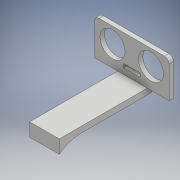
# Autodesk Inventor part: SensorMount
Saved by Autodesk Inventor 2018 (Build 220112000, 112)
## iProperties
Created: 2018-03-20
Part Number: SensorMount
Material: Generic
Document SubType Name: Modeling
Designer: reide
Density: 1 g/cm^3
Appearance: Default
Author: reide
Autodesk Inventor part; units mm, degrees
ref_plane "YZ Plane" through (0, 0, 0) normal (1, 0, 0) x (0, 1, 0)
ref_plane "XZ Plane" through (0, 0, 0) normal (0, 1, 0) x (-1, 0, 0)
ref_plane "XY Plane" through (0, 0, 0) normal (0, 0, 1) x (1, 0, 0)
sketch "Sketch1" plane through (0, 0, 0) normal (1, 0, 0) x (0, 1, 0)
  arc A0 (-24.3967, 0) -> (-49.3967, -25) centre (-24.3967, -25) ccw projected
  line L0 (-10.5765, 0) -> (-24.3967, 0) projected
  line L1 (-10.5765, 0) -> (63.7352, 0) projected
  line L2 (-24.3967, 0) -> (-39.3967, 0)
  line L3 (-39.3967, 0) -> (-39.3967, -5)
  line L4 (-39.3967, 0) -> (-3.4641, 0)
  line L5 (0, 4) -> (-39.3967, 4)
  line L6 (-39.3967, 4) -> (-39.3967, 0)
  line L7 (0, 4) -> (20, 4)
  line L8 (20, 4) -> (20, 0)
  line L9 (-3.4641, 0) -> (20, 0)
  point P0 (0, 0)
  dimension "d0" = 15
  dimension "d8" = 20
  dimension "d12" = 4
  constraints: 16 end point, 3 horizontal, 2 perpendicular, 1 collinear, 1 parallel, 1 point on circle, 1 point on line, 1 tangent
  measures "d0" distance of L0.end L2.end
  measures "d8" distance of L5.start L7.end
  measures "d12" distance of L7.end L8.end
extrude "Extrusion1" add sketch "Sketch1" along normal mid plane 20
sketch "Sketch4" plane through (-10, 20, 4) normal (0, 1, 0) x (1, 0, 0)
  line L0 (4.1911, -3.9481) -> (14.8671, -3.9481)
  line L1 (14.8671, -6.4881) -> (4.1911, -6.4881)
  line L2 (0, 0) -> (20, 0)
  line L3 (-12.5359, -24.54) -> (31.5941, -24.54)
  line L4 (34.7691, 0) -> (-15.7109, 0)
  line L5 (-15.7109, 0) -> (34.7691, 0)
  line L6 (3.9411, -6.2381) -> (3.9411, -4.1981)
  arc A0 (3.9411, -6.2381) -> (4.1911, -6.4881) centre (4.1911, -6.2381) ccw
  arc A1 (4.1911, -3.9481) -> (3.9411, -4.1981) centre (4.1911, -4.1981) ccw
  line L7 (0, 4) -> (0, 0)
  circle A2 centre (-3.4709, -13.9481) radius 8.5
  arc A3 (-15.7109, -21.365) -> (-12.5359, -24.54) centre (-12.5359, -21.365) ccw
  line L8 (-15.7109, -21.365) -> (-15.7109, 0)
  arc A4 (31.5941, -24.54) -> (34.7691, -21.365) centre (31.5941, -21.365) ccw
  line L9 (34.7691, 0) -> (34.7691, -21.365)
  line L10 (20, 0) -> (20, 4)
  line L11 (20, 4) -> (20, 2)
  arc A5 (14.8671, -6.4881) -> (15.1171, -6.2381) centre (14.8671, -6.2381) ccw
  arc A6 (15.1171, -4.1981) -> (14.8671, -3.9481) centre (14.8671, -4.1981) ccw
  circle A7 centre (22.5291, -13.9481) radius 8.5
  line L12 (15.1171, -4.1981) -> (15.1171, -6.2381)
  line L13 (0, 2) -> (0, 0)
  line L14 (0, 0) -> (20, 0)
  line L15 (20, 0) -> (20, 2)
  line L16 (0, 0) -> (20, 0) projected
  line L17 (20, 4) -> (20, 0) projected
  line L18 (20, 4) -> (0, 4) projected
  line L19 (0, 0) -> (0, 4) projected
  point P0 (10, 4)
  point P1 (10, 2)
  point P2 (10, 4)
  point P3 (10, 0)
  point P4 (10, 0)
  point P5 (24.7691, -1.4081)
  point P6 (10, 4)
  dimension "d9" = 4
  constraints: 32 end point, 12 point on circle, 8 centre point, 2 parallel, 1 horizontal, 1 midpoint, 1 point on line
  measures "d9" distance of L10.start L11.start
extrude "Extrusion3" add sketch "Sketch4" along normal blind 3
body "Solid1"
